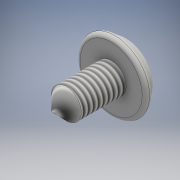
# Autodesk Inventor part: Screw
Saved by Autodesk Inventor 2016 (Build 200138000, 138)
## iProperties
Created: 2016-11-05
Part Number: Screw
Material: Generic
Document SubType Name: Modeling
Designer: Muhammad
Density: 1 g/cm^3
Appearance: Chrome - Polished
Author: Muhammad
Autodesk Inventor part; units mm, degrees
ref_plane "YZ Plane" through (0, 0, 0) normal (1, 0, 0) x (0, 1, 0)
ref_plane "XZ Plane" through (0, 0, 0) normal (0, 1, 0) x (-1, 0, 0)
ref_plane "XY Plane" through (0, 0, 0) normal (0, 0, 1) x (1, 0, 0)
sketch "Sketch1" plane through (0, 0, 0) normal (0, 1, 0) x (-1, 0, 0)
  circle A0 centre (0, 0) radius 3.5
  dimension "d0" = 7
  constraints: 1 centre point, 1 coincident
  measures "d0" diameter of A0
extrude "Extrusion1" add sketch "Sketch1" along normal blind 0.75
sketch "Sketch2" plane through (0, 0.75, 0) normal (0, 1, 0) x (1, 0, 0)
  circle A0 centre (0, 0) radius 3
  dimension "d3" = 6
  constraints: 1 centre point, 1 coincident
  measures "d3" diameter of A0
extrude "Extrusion2" add sketch "Sketch2" along normal blind 1
fillet "Fillet1" radius 1 1 edges at (-3, 1.75, 0)
fillet "Fillet2" radius 0.4 2 edges at (3.5, 0.75, 0) (3.5, 0, 0)
sketch "Sketch3" plane through (0, 0, 0) normal (0, -1, 0) x (1, 0, 0)
  circle A0 centre (0, 0) radius 1.5
  dimension "d8" = 3
  constraints: 1 centre point, 1 coincident
  measures "d8" diameter of A0
extrude "Extrusion3" add sketch "Sketch3" along normal blind 6
chamfer "Chamfer1" distance 1.5 angle 45 1 edges at (-1.5, -6, 0)
thread "Thread1" size "M3x0.5" class "6g" standard "ANSI Metric M Profile" length 10
thread "Thread2" size "R 3" standard "ISO Taper" length 10
sketch "Sketch4" plane through (0, 1.75, 0) normal (0, 1, 0) x (1, 0, 0)
  line L0 (0.5, 2) -> (-0.5, 2)
  line L1 (-0.5, 2) -> (-0.5, -2)
  line L2 (-0.5, -2) -> (0.5, -2)
  line L3 (0.5, -2) -> (0.5, 2)
  line L4 (0.5, 2) -> (-0.5, -2) construction
  line L5 (-0.5, 2) -> (0.5, -2) construction
  circle A0 centre (0, 0) radius 2 projected
  line L6 (1.9365, 0.5) -> (-1.9365, 0.5)
  line L7 (-1.9365, 0.5) -> (-1.9365, -0.5)
  line L8 (-1.9365, -0.5) -> (1.9365, -0.5)
  line L9 (1.9365, -0.5) -> (1.9365, 0.5)
  line L10 (1.9365, 0.5) -> (-1.9365, -0.5) construction
  line L11 (-1.9365, 0.5) -> (1.9365, -0.5) construction
  dimension "d18" = 1
  dimension "d19" = 4
  dimension "d20" = 1
  constraints: 24 end point, 4 midpoint, 4 parallel, 2 horizontal, 2 perpendicular, 2 other
  measures "d18" distance of L2.end L1.end
  measures "d19" distance of L1.end L0.end
  measures "d20" distance of L7.end L6.end
extrude "Extrusion4" cut sketch "Sketch4" against normal blind 0.5 contours L3 A0 L0 | A0 L1 L0 | A0 L3 L6 L1 | L6 L9 L8 L3 | L3 L8 L1 L6 | L1 L8 L7 L6 | L3 A0 L1 L8 | L3 L2 A0 | A0 L2 L1
fillet "Fillet3" radius 0.5 4 edges at (0.5, 1.5, 0.5) (0.5, 1.5, -0.5) (-0.5, 1.5, -0.5) (-0.5, 1.5, 0.5)
body "Solid1"
